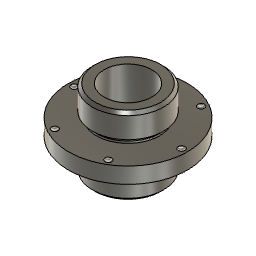
Exercise18 v4 (Autodesk Fusion 360 design; units mm, degrees)
Autodesk Fusion 360 part; units mm, degrees
sketch "Sketch1" plane through (0, 0, 0) normal (0, 1, 0) x (1, 0, 0)
  line L0 (-33.0001, 0) -> (-35.8285, -2.8284)
  line L1 (-33.0001, 0) -> (-33.002, 0) construction
  line L2 (-35.8285, -2.8284) -> (-35.8285, -23.8284)
  line L3 (-31.8323, -27.8284) -> (-31.8323, -32.0026)
  line L4 (-31.8323, -32.0026) -> (-59.8323, -32.0026)
  line L5 (-59.8323, -32.0026) -> (-59.8323, -48.0026)
  line L6 (-59.8323, -48.0026) -> (-31.8285, -48.0026)
  line L7 (-31.8285, -48.0026) -> (-31.8285, -50.0026)
  line L8 (-35.8285, -54.0026) -> (-35.8285, -75.0026)
  line L9 (-35.8285, -75.0026) -> (-33.0001, -77.8311)
  line L10 (-33.0001, -77.8311) -> (-1.0001, -77.8311)
  line L11 (-33.002, 0) -> (-1.002, 0)
  arc A0 (-35.8285, -54.0026) -> (-31.8285, -50.0026) centre (-35.8285, -50.0026) ccw
  arc A1 (-31.8323, -27.8284) -> (-35.8285, -23.8284) centre (-35.8323, -27.8284) ccw
  line L12 (-1.0001, -77.8311) -> (-1.002, 0)
  point P0 (-31.8323, -24.0026)
  point P1 (-31.8285, -54.0026)
  point P2 (-4.832, 0)
  dimension "d2" = 135
  dimension "d3" = 4
  dimension "d4" = 21
  dimension "d5" = 4
  dimension "d6" = 8
  dimension "d7" = 28
  dimension "d8" = 16
  dimension "d9" = 6
  dimension "d10" = 4
  dimension "d11" = 21
  dimension "d12" = 4
  dimension "d13" = 135
  dimension "d14" = 32
  dimension "d15" = 32
  dimension "d16" = 4
  dimension "d17" = 4
  constraint horizontal L1
  constraint vertical L2
  constraint perpendicular L3 L4
  constraint perpendicular L4 L5
  constraint perpendicular L5 L6
  constraint perpendicular L6 L7
  constraint perpendicular L6 L8
  constraint perpendicular L8 L10
  constraint perpendicular L2 L11
  constraint coincident P1 L7
  constraint tangent L7 A0
  constraint coincident L8.start A0.start
  constraint coincident P0 L3
  constraint tangent L3 A1
  constraint coincident L2.end A1.end
  constraint coincident L11 P2
  measures "d2" angle of L0 L1
  measures "d3" distance of L0.start L0.end
  measures "d4" distance of L0.end L2.end
  measures "d5" distance of L2.end P0
  measures "d6" distance of P0 L3.end
  measures "d7" distance of L3.end L4.end
  measures "d8" distance of L4.end L5.end
  measures "d9" distance of L6.end P1
  measures "d10" distance of P1 L8.start
  measures "d11" distance of L8.start L8.end
  measures "d12" distance of L8.end L9.end
  measures "d13" angle of L8 L9
  measures "d14" distance of L9.end L10.end
  measures "d15" distance of L1.end L11.end
  measures "d16" radius of A0
  measures "d17" radius of A1
revolve "Revolve1" add sketch "Sketch1" angle 360 about axis through (0, 0, 1.75) along (0, 0, 1)
sketch "Sketch2" plane through (0, 0, 77.8311) normal (0, 0, 1) x (-1, 0, 0)
  circle A0 centre (0, 0) radius 1.0001
  circle A1 centre (0, 0) radius 33.0001
  circle A2 centre (0, 0) radius 24
  dimension "d19" = 48
  constraint coincident A0.centre A1.centre
  measures "d19" diameter of A2
extrude "Extrude1" cut sketch "Sketch2" against normal blind 110 contours A2
sketch "Sketch3" plane through (0, 0, 48.0026) normal (0, 0, 1) x (-1, 0, 0)
  circle A0 centre (0, 0) radius 31.8285
  circle A1 centre (0, 0) radius 59.8323
  circle A2 centre (0, 0) radius 54
  circle A3 centre (53.999, -0.3261) radius 4
  line L0 (0, 0) -> (27, -46.7654)
  line L1 (0, 0) -> (54, 0) construction
  circle A4 centre (27, -46.7654) radius 4
  line L2 (0, 0) -> (-27, -46.7654)
  line L3 (0, 0) -> (54, 0) construction
  circle A5 centre (-27, -46.7654) radius 4
  circle A6 centre (-54, 0) radius 4
  line L4 (0, 0) -> (-27, 46.7654)
  line L5 (0, 0) -> (54, 0) construction
  line L6 (0, 0) -> (27, 46.7654)
  line L7 (0, 0) -> (54, 0) construction
  circle A7 centre (27, 46.7654) radius 4
  circle A8 centre (-27, 46.7654) radius 4
  dimension "d22" = 108
  dimension "d23" = 8
  dimension "d24" = 60
  dimension "d25" = 8
  dimension "d26" = 120
  dimension "d27" = 8
  dimension "d28" = 8
  dimension "d29" = 120
  dimension "d30" = 60
  dimension "d31" = 54
  dimension "d32" = 8
  dimension "d33" = 8
  constraint coincident A0.centre A1.centre
  constraint coincident A2 A3.centre
  constraint horizontal L1
  constraint coincident L0.end A4.centre
  constraint horizontal L3
  constraint coincident L2.end A5.centre
  constraint coincident A2 A6.centre
  constraint horizontal L5
  constraint horizontal L7
  constraint coincident L6.end A7.centre
  constraint coincident L4.end A8.centre
  measures "d22" diameter of A2
  measures "d23" diameter of A3
  measures "d24" angle of L0 L1
  measures "d25" diameter of A4
  measures "d26" angle of L2 L3
  measures "d27" diameter of A5
  measures "d28" diameter of A6
  measures "d29" angle of L4 L5
  measures "d30" angle of L6 L7
  measures "d31" distance of A0.centre L6.end
  measures "d32" diameter of A7
  measures "d33" diameter of A8
hole "Hole1" at (-54, 0, 48.0026) at (-27, 46.7654, 48.0026) at (27, 46.7654, 48.0026) at (54, 0, 48.0026) at (27, -46.7654, 48.0026) at (-27, -46.7654, 48.0026) direction (0, 0, -1) diameter 6.78 depth 15 tip angle 118
thread "Thread1" "ISO Metric profile 8.0 M8x1.25 6H" thread offset 0 thread depth 7.4
extrude "Extrude2" [suppressed]
